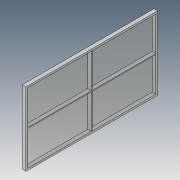
# Autodesk Inventor part: Window
Saved by Autodesk Inventor 2018.3 (Build 223284000, 284)
## iProperties
Created: 2019-11-07
Part Number: Window
Material: Generic
Document SubType Name: Modeling
Designer: MattBussey
Density: 1 g/cm^3
Appearance: Default
Author: MattBussey
Autodesk Inventor part; units mm, degrees
ref_plane "YZ Plane" through (0, 0, 0) normal (1, 0, 0) x (0, 1, 0)
ref_plane "XZ Plane" through (0, 0, 0) normal (0, 1, 0) x (-1, 0, 0)
ref_plane "XY Plane" through (0, 0, 0) normal (0, 0, 1) x (1, 0, 0)
sketch "Sketch1" plane through (0, 0, 0) normal (1, 0, 0) x (0, 1, 0)
  line L0 (0, 0) -> (508, 0)
  line L1 (508, 0) -> (508, -914.4)
  line L2 (508, -914.4) -> (0, -914.4)
  line L3 (0, -914.4) -> (0, 0)
  line L4 (495.3, -901.7) -> (495.3, -12.7)
  line L5 (495.3, -12.7) -> (12.7, -12.7)
  line L6 (12.7, -12.7) -> (12.7, -901.7)
  line L7 (12.7, -901.7) -> (495.3, -901.7)
  line L8 (495.3, -12.7) -> (257.175, -12.7)
  line L9 (257.175, -12.7) -> (257.175, -454.025)
  line L10 (257.175, -454.025) -> (495.3, -454.025)
  line L11 (495.3, -454.025) -> (495.3, -12.7)
  line L12 (495.3, -901.7) -> (257.175, -901.7)
  line L13 (257.175, -901.7) -> (257.175, -460.375)
  line L14 (257.175, -460.375) -> (495.3, -460.375)
  line L15 (495.3, -460.375) -> (495.3, -901.7)
  line L16 (12.7, -901.7) -> (250.825, -901.7)
  line L17 (250.825, -901.7) -> (250.825, -460.375)
  line L18 (250.825, -460.375) -> (12.7, -460.375)
  line L19 (12.7, -460.375) -> (12.7, -901.7)
  line L20 (12.7, -12.7) -> (250.825, -12.7)
  line L21 (250.825, -12.7) -> (250.825, -454.025)
  line L22 (250.825, -454.025) -> (12.7, -454.025)
  line L23 (12.7, -454.025) -> (12.7, -12.7)
  dimension "d0" = 914.4
  dimension "d1" = 508
  dimension "d3" = 12.7
  dimension "d4" = 6.35
  dimension "d5" = 6.35
  constraints: 48 end point, 12 parallel, 6 equal length, 6 perpendicular, 5 horizontal, 3 other
  measures "d0" distance of L0.end L1.end
  measures "d1" distance of L0.start L0.end
  measures "d3" distance between parallel lines of L1 L4
  measures "d4" distance between parallel lines of L21 L9
  measures "d5" distance between parallel lines of L14 L10
extrude "Extrusion1" add sketch "Sketch1" along normal blind 25.4 contours L7 L13 L14 L4 | L10 L9 L5 L4 | L7 L6 L18 L17 | L21 L22 L6 L5
extrude "Extrusion2" add sketch "Sketch1" along normal blind 25.4 separate body contours L0 L1 L2 L3 | L14 L13 L7 L17 L18 L6 L22 L21 L5 L9 L10 L4
equation "\"d5\" = d4"
